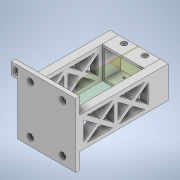
# Autodesk Inventor part: 부품4
Saved by Autodesk Inventor 2020 (Build 240168000, 168)
## iProperties
Created: 2019-09-25
Part Number: 부품4
Material: 일반
Document SubType Name: Modeling
Designer: Knowblesse
Density: 1 g/cm^3
Appearance: 기본값
Author: Knowblesse
## iProperties of the stored document _3D 인쇄.ipt
Created: 2019-09-26
Part Number: _3D 인쇄
Material: 일반
Document SubType Name: Modeling
Designer: Knowblesse
Density: 1 g/cm^3
Appearance: 기본값
Author: Knowblesse
Autodesk Inventor part; units mm, degrees
ref_plane "YZ Plane" through (0, 0, 0) normal (1, 0, 0) x (0, 1, 0)
ref_plane "XZ Plane" through (0, 0, 0) normal (0, 1, 0) x (-1, 0, 0)
ref_plane "XY Plane" through (0, 0, 0) normal (0, 0, 1) x (1, 0, 0)
sketch "스케치1" plane through (0, 0, 0) normal (0, 0, 1) x (1, 0, 0)
  line L0 (0, 0) -> (46, 0)
  line L1 (46, 0) -> (46, 33.5)
  line L2 (46, 33.5) -> (0, 33.5)
  line L3 (0, 33.5) -> (0, 0)
  line L4 (-3, 36.5) -> (49, 36.5)
  line L5 (49, 36.5) -> (49, -3)
  line L6 (49, -3) -> (-3, -3)
  line L7 (-3, -3) -> (-3, 36.5)
  dimension "d0" = 46
  dimension "d1" = 33.5
  dimension "t" = 3
  constraints: 16 end point, 4 parallel, 2 perpendicular, 1 horizontal, 3 other
  measures "d0" distance of L2.end L1.end
  measures "d1" distance of L1.end L0.end
  measures "t" distance between parallel lines of L2 L4
extrude "돌출1" add sketch "스케치1" along normal blind 20
sketch "스케치3" plane through (-3, -3, 0) normal (0, -1, 0) x (1, 0, 0)
  line L0 (0, 0) -> (0, 20) projected
  line L1 (52, 0) -> (52, 20) projected
  line L2 (0, 0) -> (52, 0) projected
  point P0 (3, 0)
  point P1 (13, 6)
  point P2 (39, 6)
  dimension "d17" = 26
  dimension "d18" = 13
  dimension "d19" = 13
  dimension "d60" = 6
  constraints: 1 horizontal alignment
  measures "d17" distance of point (39, 6) point (13, 6)
  measures "d18" distance from line of L0 point (13, 6)
  measures "d19" distance from line of L1 point (39, 6)
  measures "d60" distance from line of point (13, 6) L2
hole "구멍1" at (10, -3, 6) at (36, -3, 6) direction (0, 1, 0) diameter 3 depth 3 counterbore diameter 7 counterbore depth 2
ref_plane "작업 평면1" through (-3, 16.75, 0) normal (0, 1, 0) x (1, 0, 0)
mirror "미러1" about plane through (-3, 16.75, 0) normal (0, 1, 0) of "구멍1"
sketch "스케치4" plane through (49, -3, 0) normal (1, 0, 0) x (0, 0, -1)
  line L0 (0, 0) -> (0, 39.5) projected
  line L1 (0, 39.5) -> (-20, 39.5) projected
  line L2 (-20, 0) -> (-20, 39.5) projected
  line L3 (0, 0) -> (-20, 0) projected
  point P0 (0, 3)
extrude "돌출3" add sketch "스케치4" along normal blind 5 separate body
sketch "스케치6" plane through (54, -3, 0) normal (1, 0, 0) x (0, 0, -1)
  line L0 (0, 0) -> (-20, 0) projected
  line L1 (0, 0) -> (-110, 0)
  line L2 (-110, 0) -> (-110, 39.5)
  line L3 (-110, 39.5) -> (0, 39.5)
  line L4 (0, 39.5) -> (0, 0)
  line L5 (0, 39.5) -> (-20, 39.5) projected
  line L6 (-20, 39.5) -> (-20, 0) projected
  line L7 (-20, 39.5) -> (-110, 39.5)
  line L8 (-110, 39.5) -> (-110, 0)
  line L9 (-110, 0) -> (-20, 0)
  line L10 (-20, 0) -> (-20, 39.5)
  line L11 (-25, 5) -> (-105, 5)
  line L12 (-105, 5) -> (-105, 34.5)
  line L13 (-105, 34.5) -> (-25, 34.5)
  line L14 (-25, 34.5) -> (-25, 5)
  line L15 (-25, 5) -> (-65, 34.5)
  line L16 (-105, 5) -> (-65, 34.5)
  line L17 (-66.4839, 36.512) -> (-106.4839, 7.012)
  line L18 (-106.4839, 7.012) -> (-103.5161, 2.988)
  line L19 (-103.5161, 2.988) -> (-63.5161, 32.488)
  line L20 (-63.5161, 32.488) -> (-66.4839, 36.512)
  line L21 (-66.4839, 36.512) -> (-103.5161, 2.988) construction
  line L22 (-106.4839, 7.012) -> (-63.5161, 32.488) construction
  line L23 (-66.4839, 32.488) -> (-26.4839, 2.988)
  line L24 (-26.4839, 2.988) -> (-23.5161, 7.012)
  line L25 (-23.5161, 7.012) -> (-63.5161, 36.512)
  line L26 (-63.5161, 36.512) -> (-66.4839, 32.488)
  line L27 (-66.4839, 32.488) -> (-23.5161, 7.012) construction
  line L28 (-26.4839, 2.988) -> (-63.5161, 36.512) construction
  line L29 (-67.5, 34.5) -> (-67.5, 5)
  line L30 (-67.5, 5) -> (-62.5, 5)
  line L31 (-62.5, 5) -> (-62.5, 34.5)
  line L32 (-62.5, 34.5) -> (-67.5, 34.5)
  line L33 (-67.5, 34.5) -> (-62.5, 5) construction
  line L34 (-67.5, 5) -> (-62.5, 34.5) construction
  line L35 (-63.5161, 7.012) -> (-103.5161, 36.512)
  line L36 (-103.5161, 36.512) -> (-106.4839, 32.488)
  line L37 (-106.4839, 32.488) -> (-66.4839, 2.988)
  line L38 (-66.4839, 2.988) -> (-63.5161, 7.012)
  line L39 (-63.5161, 7.012) -> (-106.4839, 32.488) construction
  line L40 (-103.5161, 36.512) -> (-66.4839, 2.988) construction
  line L41 (-26.4839, 36.512) -> (-66.4839, 7.012)
  line L42 (-66.4839, 7.012) -> (-63.5161, 2.988)
  line L43 (-63.5161, 2.988) -> (-23.5161, 32.488)
  line L44 (-23.5161, 32.488) -> (-26.4839, 36.512)
  line L45 (-26.4839, 36.512) -> (-63.5161, 2.988) construction
  line L46 (-66.4839, 7.012) -> (-23.5161, 32.488) construction
  point P0 (0, 3)
  point P1 (-85, 19.75)
  point P2 (-45, 19.75)
  point P3 (-65, 34.5)
  point P4 (-69.212, 34.5)
  point P5 (-105, 8.1064)
  point P6 (-25, 8.1064)
  point P7 (-60.788, 34.5)
  point P8 (-65, 31.3936)
  point P9 (-29.212, 5)
  point P10 (-100.788, 5)
  point P11 (-65, 19.75)
  point P12 (-105, 19.75)
  point P13 (-65, 19.75)
  point P14 (-65, 19.75)
  point P15 (-65, 5)
  point P16 (-62.5, 5)
  point P17 (-62.5, 29.5499)
  point P18 (-67.5, 29.5499)
  point P19 (-67.5, 5)
  point P20 (-65, 34.5)
  point P21 (-49.212, 19.75)
  point P22 (-62.5, 9.9501)
  point P23 (-67.5, 9.9501)
  point P24 (-80.788, 19.75)
  point P25 (-105, 31.3936)
  point P26 (-89.212, 19.75)
  point P27 (-85, 16.6436)
  point P28 (-69.212, 5)
  point P29 (-29.212, 34.5)
  point P30 (-45, 22.8564)
  point P31 (-40.788, 19.75)
  point P32 (-25, 31.3936)
  point P33 (-45, 16.6436)
  point P34 (-60.788, 5)
  point P35 (-85, 22.8564)
  point P36 (-100.788, 34.5)
  dimension "d22" = 110
  dimension "d23" = 5
  dimension "d24" = 5
  dimension "d25" = 5
  dimension "d28" = 5
  dimension "d64" = 5
  dimension "d65" = 5
  constraints: 88 end point, 22 midpoint, 18 parallel, 8 perpendicular, 2 collinear, 2 horizontal, 1 horizontal alignment, 1 vertical alignment, 3 other
  measures "d22" distance of L2.end L3.end
  measures "d23" distance between parallel lines of L9 L11
  measures "d24" distance of L18.end L17.end
  measures "d25" distance of L24.end L23.end
  measures "d28" distance of L30.end L29.end
  measures "d64" distance of L36.end L35.end
  measures "d65" distance of L42.end L41.end
extrude "돌출4" add sketch "스케치6" along normal mid plane 10 contours L0 L6 L3 L4 | L1 L2 L3 L6 | L24 L23 L11 | L15 L43 L25 L14 | L11 L23 L43 L15 | L14 L25 L24 | L43 L23 L41 L15 | L15 L41 L25 L43 | L43 L42 L11 | L11 L31 L41 L23 L43 | L43 L25 L41 L13 L14 | L14 L44 L43 | L41 L23 L31 L15 | L15 L31 L13 L25 L41 | L11 L38 L35 L41 L31 | L13 L41 L44 | L31 L23 L19 L20 L15 | L15 L13 L31 | L38 L37 L11 | L42 L41 L35 L38 | L11 L29 L35 L41 L42 | L41 L35 L29 L19 L23 L31 | L13 L26 L25 | L16 L29 L13 | L26 L23 L19 L29 L16 | L13 L17 L20 | L20 L19 L23 L26 | L11 L37 L19 L35 L29 | L29 L16 L35 L17 L13 | L29 L19 L35 L16 | L35 L19 L37 L16 | L16 L37 L17 L35 | L19 L18 L11 | L11 L16 L37 L19 | L35 L17 L37 L12 L13 | L13 L36 L35 | L16 L12 L17 L37 | L18 L17 L12 | L12 L37 L36 bodies 2
ref_plane "작업 평면2" through (23, 0, 20) normal (-1, 0, 0) x (0, 0, 1)
mirror "미러2" about plane through (23, 0, 20) normal (-1, 0, 0) of "돌출3", "돌출4" bodies 2
sketch "스케치12" plane through (49, -3, 110) normal (0, 0, 1) x (1, 0, 0)
  line L0 (10, 59.5) -> (-62, 59.5)
  line L1 (-62, 59.5) -> (-62, -20)
  line L2 (-62, -20) -> (10, -20)
  line L3 (10, -20) -> (10, 59.5)
  line L4 (10, 39.5) -> (10, 0) projected
  line L5 (-62, 39.5) -> (-62, 0) projected
  line L6 (0, 39.5) -> (-52, 39.5) projected
  line L7 (-52, 0) -> (0, 0) projected
  dimension "d71" = 20
  dimension "d72" = 20
  constraints: 8 end point, 2 collinear, 2 parallel, 1 horizontal, 1 perpendicular
  measures "d71" distance between parallel lines of L0 L6
  measures "d72" distance between parallel lines of L2 L7
extrude "돌출8" add sketch "스케치12" along normal blind 5 bodies 2
sketch "스케치13" plane through (49, -3, 110) normal (0, 0, -1) x (-1, 0, 0)
  line L0 (62, 0) -> (62, -20) projected
  line L1 (-10, -20) -> (-10, 0) projected
  line L2 (62, 59.5) -> (62, 39.5) projected
  point P0 (49, 3)
  point P1 (46, -10)
  point P2 (6, -10)
  point P3 (6, 49.5)
  point P4 (46, 49.5)
  point P5 (62, -10)
  point P6 (62, 49.5)
  dimension "d73" = 40
  dimension "d74" = 16
  dimension "d75" = 16
  constraints: 4 horizontal alignment, 2 midpoint, 2 vertical alignment
  measures "d73" distance of point (6, -10) point (46, -10)
  measures "d74" distance from line of L0 point (46, -10)
  measures "d75" distance from line of L1 point (6, -10)
hole "구멍4" at (3, -13, 110) at (43, -13, 110) at (43, 46.5, 110) at (3, 46.5, 110) direction (0, 0, 1) diameter 8 end through all bodies 2
sketch "스케치14" plane through (49, -3, 115) normal (0, 0, 1) x (1, 0, 0)
  line L0 (-62, 59.5) -> (-62, -20) projected
  line L1 (-62, 59.5) -> (-70, 59.5)
  line L2 (-70, 59.5) -> (-70, 44.5)
  line L3 (-70, 44.5) -> (-62, 44.5)
  line L4 (-62, 44.5) -> (-62, 59.5)
  line L5 (-62, 48) -> (-67, 48)
  line L6 (-67, 48) -> (-67, 56)
  line L7 (-67, 56) -> (-62, 56)
  line L8 (-62, 56) -> (-62, 48)
  point P0 (-49, 3)
  dimension "d83" = 8
  dimension "d84" = 15
  dimension "d85" = 5
  dimension "d86" = 8
  dimension "d87" = 3.5
  dimension "d88" = 3.5
  constraints: 16 end point, 4 parallel, 2 horizontal, 2 perpendicular, 1 point on line
  measures "d83" distance of L3.end L2.end
  measures "d84" distance of L2.end L1.end
  measures "d85" distance of L6.end L7.end
  measures "d86" distance of L5.end L6.end
  measures "d87" distance between parallel lines of L1 L7
  measures "d88" distance between parallel lines of L3 L5
extrude "돌출9" add sketch "스케치14" against normal blind 5 contours L0 L7 L6 L5 L3 L2 L1 bodies 2
equation "\"d18\" = d19"
equation "\"d74\" = d75"
equation "\"d87\" = d88"
